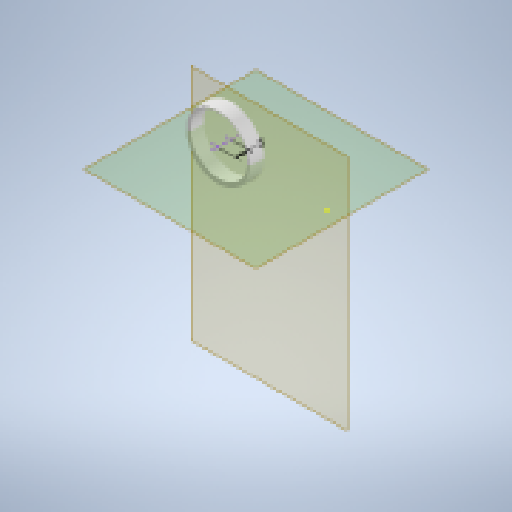
# Autodesk Inventor part: Aeration
Saved by Autodesk Inventor 2023 (Build 270158000, 158)
## iProperties
Created: 2023-03-27
Part Number: Aeration
Material: Générique
Document SubType Name: Modeling
Designer: eleves
Density: 1 g/cm^3
Appearance: Par défaut
Author: eleves
Autodesk Inventor part; units mm, degrees
ref_plane "YZ Plane" through (0, 0, 0) normal (1, 0, 0) x (0, 1, 0)
ref_plane "XZ Plane" through (0, 0, 0) normal (0, 1, 0) x (-1, 0, 0)
ref_plane "XY Plane" through (0, 0, 0) normal (0, 0, 1) x (1, 0, 0)
sketch "Esquisse1" plane through (0, 0, 0) normal (0, 0, 1) x (1, 0, 0)
  circle A0 centre (-41.5, 69.6) radius 12.5 projected
  circle A1 centre (-41.5, 69.6) radius 11
  circle A2 centre (-41.5, 69.6) radius 13
  point P0 (0, 0)
  dimension "d11" = 0.5
  dimension "d15" = 2
  constraints: 2 centre point
  measures "d11" radial gap between concentric circles of A0 A2
  measures "d15" radial gap between concentric circles of A1 A2
ref_plane "Plan de construction2" through (-41.5, 69.6, 0) normal (0, -1, 0) x (0, 0, 1)
ref_plane "Plan de construction1" through (0, 0, -152.2) normal (0, -1, 0) x (0, 0, 1)
sketch "Esquisse2" plane through (-41.5, 69.6, 0) normal (0, -1, 0) x (0, 0, 1)
  point P0 (0, -41.5)
  point P1 (0, 0)
  point P2 (-5, 0)
  dimension "d1" = 5
  measures "d1" distance of point (0, 0) point (-5, 0)
ref_plane "Plan de construction4" through (-41.5, 69.6, -5) normal (0, 0, 1) x (1, 0, 0)
ref_plane "Plan de construction3" through (0, 0, 0) normal (0, 0, 1) x (1, 0, 0)
sketch "Esquisse3" plane through (-41.5, 69.6, -5) normal (0, 0, 1) x (1, 0, 0)
  circle A0 centre (0, 0) radius 12.5 projected
  circle A1 centre (0, 0) radius 9.5
  circle A2 centre (0, 0) radius 11.5
  point P0 (41.5, -69.6)
  dimension "d13" = 2
  dimension "d14" = 1
  constraints: 2 centre point
  measures "d13" radial gap between concentric circles of A2 A1
  measures "d14" radial gap between concentric circles of A0 A2
ref_plane "Plan de construction5" through (-41.5, 69.6, 0) normal (0, 0, 1) x (1, 0, 0)
loft "Lissage2" add profiles "Esquisse3", "Esquisse1" contours A1 | A2 / A0 | A1 | A2
sketch "Esquisse5" plane through (-41.5, 69.6, 0) normal (0, 0, 1) x (1, 0, 0)
  circle A0 centre (0.1842, -0.128) radius 10.7757
  circle A1 centre (0, 0) radius 13 projected
  point P0 (41.5, -69.6)
  dimension "d20" = 2
  constraints: 1 centre point
extrude "Extrusion2" cut sketch "Esquisse5" against normal blind 10 contours A0
ref_plane "Plan de construction6" through (0, 0, 0) normal (-1, 0, 0) x (0, -1, 0)
sketch "Esquisse6" plane through (0, 0, 0) normal (-1, 0, 0) x (0, -1, 0)
  point P0 (0, 0)
sketch "Esquisse7" plane through (-41.5, 69.6, 0) normal (0, 0, 1) x (1, 0, 0)
  circle A0 centre (0.1842, -0.128) radius 10.7757 projected
  circle A1 centre (0, 0) radius 13 projected
  point P0 (41.5, -69.6)
sketch "Esquisse8" plane through (0, 0, 0) normal (-1, 0, 0) x (0, -1, 0)
  line L0 (0, 5) -> (-101.6415, 5)
  point P0 (0, 0)
  dimension "d23" = 5
  constraints: 2 end point, 1 horizontal
  measures "d23" distance from line of point (0, 0) L0
revolve "Révolution1" add sketch "Esquisse7" angle 90 about axis through (0, 0, 5) along (0, 1, 0)
sketch "Esquisse9" plane through (-5, 69.6, 46.5) normal (1, 0, 0) x (0, 0, -1)
  circle A0 centre (0, 0) radius 13 projected
  circle A1 centre (0.1842, -0.128) radius 10.7757 projected
  point P0 (46.5, -69.6)
  point P1 (13, 0)
  point P2 (10.9599, -0.128)
  constraints: 2 horizontal alignment
extrude "Extrusion3" add sketch "Esquisse9" along normal up to surface (5 mm away)
sketch "Esquisse10" plane through (0, 69.6, 46.5) normal (1, 0, 0) x (0, 0, -1)
  circle A0 centre (0.1842, -0.128) radius 10.7757 projected
  line L0 (2.1644, -3.5577) -> (-1.7959, -3.5577)
  line L1 (-1.7959, -3.5577) -> (-3.7761, -0.128)
  line L2 (-3.7761, -0.128) -> (-1.7959, 3.3017)
  line L3 (-1.7959, 3.3017) -> (2.1644, 3.3017)
  line L4 (2.1644, 3.3017) -> (4.1445, -0.128)
  line L5 (4.1445, -0.128) -> (2.1644, -3.5577)
  line L6 (2.4473, -3.0677) -> (6.2069, -9.0635)
  line L7 (1.5742, -3.5577) -> (5.3525, -9.5834)
  line L8 (3.8616, 0.362) -> (10.9339, 0.62)
  line L9 (3.8494, -0.6391) -> (10.9569, -0.3798)
  line L10 (1.5986, 3.3017) -> (4.9112, 9.5555)
  line L11 (2.4595, 2.7906) -> (5.7886, 9.0755)
  line L12 (-2.0788, 2.8117) -> (-5.8384, 8.8074)
  line L13 (-1.2058, 3.3017) -> (-4.9841, 9.3273)
  line L14 (-3.4932, -0.618) -> (-10.5654, -0.8761)
  line L15 (-3.481, 0.3831) -> (-10.5885, 0.1237)
  line L16 (-1.2301, -3.5577) -> (-4.5428, -9.8115)
  line L17 (-2.091, -3.0466) -> (-5.4202, -9.3316)
  point P0 (46.5, -69.6)
  point P1 (3.8494, -0.6391)
  point P2 (10.9569, -0.3798)
  point P3 (10.9339, 0.62)
  point P4 (3.8616, 0.362)
  point P5 (2.4595, 2.7906)
  point P6 (5.7886, 9.0755)
  point P7 (4.9112, 9.5555)
  point P8 (1.5986, 3.3017)
  point P9 (-1.2058, 3.3017)
  point P10 (-4.9841, 9.3273)
  point P11 (-5.8384, 8.8074)
  point P12 (-2.0788, 2.8117)
  point P13 (-3.481, 0.3831)
  point P14 (-10.5885, 0.1237)
  point P15 (-10.5654, -0.8761)
  point P16 (-3.4932, -0.618)
  point P17 (-2.091, -3.0466)
  point P18 (-5.4202, -9.3316)
  point P19 (-4.5428, -9.8115)
  point P20 (-1.2301, -3.5577)
  dimension "d28" = 0.5
  dimension "d29" = 0.5
  dimension "d32" = 360
  constraints: 36 end point, 2 point on circle, 2 point on line, 1 coincident, 1 horizontal, 1 parallel, 50 other
  measures "d28" distance from line of L0.start L6
  measures "d29" distance from line of L0.start L7
extrude "Extrusion4" add sketch "Esquisse10" against normal blind 2 contours A0 L9 L5 L4 L8 | L11 L4 L3 L10 A0 | L4 L5 L0 L1 L2 L3 | A0 L7 L0 L5 L6 | L13 L3 L2 L12 A0 | A0 L17 L1 L0 L16 | L15 L2 L1 L14 A0
